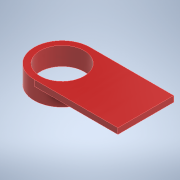
# Autodesk Inventor part: bottomAttachementForPvcPipe
Saved by Autodesk Inventor 2022.2 (Build 262287000, 287)
## iProperties
Created: 2021-10-20
Part Number: bottomAttachementForPvcPipe
Material: PC/ABS Plastic
Document SubType Name: Modeling
Designer: robst
Density: 0.357273 g/cm^3
Appearance: Red
Author: robst
Autodesk Inventor part; units mm, degrees
ref_plane "YZ Plane" through (0, 0, 0) normal (1, 0, 0) x (0, 1, 0)
ref_plane "XZ Plane" through (0, 0, 0) normal (0, 1, 0) x (-1, 0, 0)
sketch "Sketch61" plane through (0, 0, 0) normal (0, 1, 0) x (-1, 0, 0)
  circle A0 centre (0, 0) radius 30.1625
  circle A1 centre (0, 0) radius 38.1625
  dimension "d320" = 60.325
  dimension "d321" = 8
  constraints: 2 centre point, 2 coincident
  measures "d320" diameter of A0
  measures "d321" radial gap between concentric circles of A1 A0
extrude "Extrusion30" add sketch "Sketch61" along normal mid plane 25
sketch "Sketch62" plane through (0, 12.5, 0) normal (0, 1, 0) x (1, 0, 0)
  circle A0 centre (0, 0) radius 38.1625 projected
  line L0 (0, 38.1625) -> (114.3625, 38.1625)
  line L1 (114.3625, 38.1625) -> (114.3625, 0)
  line L2 (0, -38.1625) -> (114.3625, -38.1625)
  line L3 (114.3625, -38.1625) -> (114.3625, 0)
  dimension "d325" = 76.2
  constraints: 8 end point, 3 perpendicular, 2 point on circle, 1 collinear, 1 horizontal, 1 point on line, 1 tangent
  measures "d325" distance edge to line of A0 L1
extrude "Extrusion31" add sketch "Sketch62" against normal blind 8 contours A0 L0 L1 L3 L2
sketch "Sketch51" plane through (0, 0, 0) normal (0, 1, 0) x (-1, 0, 0)
  circle A0 centre (0, 0) radius 57.15
  dimension "d242" = 114.3
  constraints: 1 centre point, 1 coincident
  measures "d242" diameter of A0
sketch "Sketch58" plane through (0, 0, 0) normal (0, 1, 0) x (1, 0, 0)
  circle A0 centre (0, 0) radius 31.4309 construction
  point P0 (0, 47.625)
  point P1 (-23.8125, 41.2445)
  point P2 (-41.2445, 23.8125)
  point P3 (-47.625, 0)
  point P4 (-41.2445, -23.8125)
  point P5 (-23.8125, -41.2445)
  point P6 (0, -47.625)
  point P7 (23.8125, -41.2445)
  point P8 (41.2445, -23.8125)
  point P9 (47.625, 0)
  point P10 (41.2445, 23.8125)
  point P11 (23.8125, 41.2445)
  dimension "d294" = 47.625
  dimension "d297" = 360
  constraints: 1 centre point, 13 other
  measures "d294" distance of point (0, 47.625) point (0, 0)
sketch "Sketch59" plane through (0, -8, 0) normal (0, -1, 0) x (1, 0, 0)
  circle A0 centre (0, 0) radius 38.1
  circle A1 centre (0, 0) radius 28.575
  dimension "d306" = 76.2
  dimension "d307" = 9.525
  constraints: 2 centre point, 2 coincident
  measures "d306" diameter of A0
  measures "d307" radial gap between concentric circles of A1 A0
sketch "Sketch60" plane through (0, -8, 38.1) normal (0, 0, 1) x (1, 0, 0)
  line L0 (-38.1, -35) -> (38.1, -35) projected
  line L1 (-57.15, 0) -> (57.15, 0) projected
  line L2 (38.1, 0) -> (38.1, -35) projected
  line L3 (-38.1, 0) -> (-38.1, -35) projected
  line L4 (-28.575, 0) -> (28.575, 0) construction
  line L5 (0, 0) -> (0, -35) construction
  line L6 (28.575, -35) -> (-28.575, -35) construction
  point P0 (0, 8)
  point P1 (0, -17.5)
  constraints: 3 midpoint, 2 end point
equation "\"d242\" = outsideDiameterOfPart"
equation "\"d306\" = insideDiameterOfPipe"
equation "\"wallThickness\" = 8"
equation "\"twoByFourWidth\" = 40.64"
equation "\"twoByFourDepth\" = 84.1375"
equation "\"azimuth\" = 55deg"
equation "\"elevationOfTwoByFour\" = 20deg"
equation "\"depthOfExtrusionForMatingToLowerHalf\" = 12.5"
equation "\"depthForWasherForMatingToCase\" = 14"
equation "\"pvc2InchPipeInsideDiameter\" = 52.5018"
equation "\"pvc2InchPipeOutsideDiameter\" = 60.325"
equation "\"pvcPipeInsertDepth\" = 25"
equation "\"outsideDiameterOfPipe\" = 88.9"
equation "\"insideDiameterOfPipe\" = 76.2"
equation "\"outsideDiameterOfPart\" = 114.3"
equation "\"pvc3InchPipeOutsideDiameter\" = 88.9"
body "Solid4"
body "Solid5"
